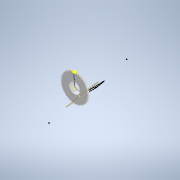
# Autodesk Inventor part: BigGear54T
Saved by Autodesk Inventor 2022 (Build 260153070, 153G)
## iProperties
Created: 2021-11-03
Part Number: BigGear54T
Material: Generic
Document SubType Name: Modeling
Designer: a laptop
Density: 1 g/cm^3
Appearance: Default
Author: a laptop
Autodesk Inventor part; units mm, degrees
ref_plane "YZ Plane" through (0, 0, 0) normal (1, 0, 0) x (0, 1, 0)
ref_plane "XZ Plane" through (0, 0, 0) normal (0, 1, 0) x (-1, 0, 0)
ref_plane "XY Plane" through (0, 0, 0) normal (0, 0, 1) x (1, 0, 0)
sketch "Sketch1" plane through (0, 0, 0) normal (0, 0, 1) x (1, 0, 0)
  spline S0 degree 3 poles (-1.174, 28.63) (-1.0927, 28.4349) (-0.9299, 28.0448) (-0.6964, 27.4567) (-0.6845, 26.9812) (-0.5323, 26.7628) (-0.4495, 26.6948) (-0.2625, 26.656) (0, 26.6828) (0.2625, 26.656) (0.4495, 26.6948) (0.5323, 26.7628) (0.6845, 26.9812) (0.6964, 27.4567) (0.9299, 28.0448) (1.0927, 28.4349) (1.174, 28.63) knots 0 0 0 0 0.063388 0.126771 0.190074 0.197992 0.205919 0.221604 0.2533 0.284997 0.300682 0.308609 0.316526 0.37983 0.443213 0.506601 0.506601 0.506601 0.506601
  circle A0 centre (0, 0) radius 26.6721 construction
  circle A1 centre (0, 0) radius 26.5898 construction
  circle A2 centre (0, 0) radius 27 construction
  circle A3 centre (0, 0) radius 28.654
  point P0 (-0.9317, 28.0443)
  point P1 (-0.7324, 27.4425)
  point P2 (-0.5764, 26.829)
  point P3 (-0.5295, 26.7652)
  point P4 (-0.4679, 26.7154)
  point P5 (-0.317, 26.6726)
  point P6 (0, 26.6721)
  point P7 (0.317, 26.6726)
  point P8 (0.4679, 26.7154)
  point P9 (0.5295, 26.7652)
  point P10 (0.5764, 26.829)
  point P11 (0.7324, 27.4425)
  point P12 (0.9317, 28.0443)
  constraints: 4 centre point, 2 point on circle, 35 other
extrude "Extrusion1" add sketch "Sketch1" against normal blind 3
extrude "Extrusion2" cut sketch "Sketch1" against normal blind 10 contours A3 S0 picked at (-0.134, 28.0575)
pattern_circular "Circular Pattern1" count 54 over 360 about axis through (0, 0, 0) along (0, 0, -1) of "Extrusion2"
sketch "Sketch2" plane through (0, 0, 0) normal (0, 0, 1) x (1, 0, 0)
  spline S0 degree 3 poles (-1.174, 28.63) (-1.0927, 28.4349) (-0.9299, 28.0448) (-0.6964, 27.4567) (-0.6845, 26.9812) (-0.5323, 26.7628) (-0.4495, 26.6948) (-0.2625, 26.656) (0, 26.6828) (0.2625, 26.656) (0.4495, 26.6948) (0.5323, 26.7628) (0.6845, 26.9812) (0.6964, 27.4567) (0.9299, 28.0448) (1.0927, 28.4349) (1.174, 28.63) knots 0 0 0 0 0.063388 0.126771 0.190074 0.197992 0.205919 0.221604 0.2533 0.284997 0.300682 0.308609 0.316526 0.37983 0.443213 0.506601 0.506601 0.506601 0.506601 projected
  arc A0 (-1.174, 28.63) -> (-2.1576, 28.5727) centre (0, 0) ccw projected
  line L0 (-2.1576, 28.5727) -> (-1.6658, 28.6013) construction
  arc A1 (2.1576, 28.5727) -> (1.174, 28.63) centre (0, 0) ccw projected
  line L1 (-1.174, 28.63) -> (0, 28.63) construction
  line L2 (-1.6658, 28.6013) -> (0, 0) construction
  line L3 (0, 28.63) -> (0, 0) construction
  line L4 (0, 28.63) -> (1.174, 28.63) construction
  line L5 (-1.6658, 28.6013) -> (-1.174, 28.63) construction
  constraints: 12 end point, 3 perpendicular, 2 horizontal, 1 coincident, 1 collinear, 1 other
sketch "Sketch3" plane through (0, 0, 0) normal (0, 0, 1) x (1, 0, 0)
  circle A0 centre (0, 0) radius 11.05
  circle A1 centre (0, 0) radius 14.05
  dimension "d7" = 22.1
  dimension "d8" = 3
  constraints: 2 centre point, 2 coincident
  measures "d7" diameter of A0
  measures "d8" radial gap between concentric circles of A1 A0
extrude "Extrusion3" add sketch "Sketch3" against normal blind 9.5
sketch "Sketch4" plane through (0, 0, -9.5) normal (0, 0, -1) x (-1, 0, 0)
  circle A0 centre (0, 0) radius 14.05 projected
  circle A1 centre (0, 0) radius 9.3
  circle A2 centre (0, 0) radius 11.05 construction
  dimension "d11" = 1.75
  constraints: 1 centre point, 1 coincident
  measures "d11" radial gap between concentric circles of A2 A1
extrude "Extrusion4" add sketch "Sketch4" along normal blind 1.5
extrude "Extrusion5" cut sketch "Sketch3" against normal blind 3 contours A0
ref_plane "Work Plane1" through (26.7535, 10.2617, 0) normal (0.7699292, -0.6381293, 0) x (0.6381293, 0.7699292, 0)
sketch "Sketch5" plane through (26.7535, 10.2617, 0) normal (0.7699292, -0.6381293, 0) x (0.6381293, 0.7699292, 0)
  line L0 (-10.923, -3) -> (-39.023, -3) projected
  line L1 (-24.973, -3) -> (-24.973, -43.285) construction
  line L2 (-12.973, -3) -> (-12.973, -16.8196)
  circle A0 centre (-13.603, -40.285) radius 1.5
  circle A1 centre (-13.603, -40.285) radius 3
  arc A2 (-12.973, -16.8196) -> (-10.6636, -39.6851) centre (101.378, -16.8196) ccw
  line L3 (-13.603, -43.285) -> (-24.973, -43.285)
  line L4 (-36.973, -3) -> (-36.973, -16.8196)
  circle A3 centre (-36.343, -40.285) radius 1.5
  circle A4 centre (-36.343, -40.285) radius 3
  arc A5 (-39.2824, -39.6851) -> (-36.973, -16.8196) centre (-151.3239, -16.8196) ccw
  line L5 (-36.343, -43.285) -> (-24.973, -43.285)
  point P0 (-24.973, 0)
  dimension "d16" = 3
  dimension "d17" = 1.5
  dimension "d18" = 12
  dimension "d19" = 26.4654
  constraints: 10 end point, 8 point on circle, 7 symmetric about line, 6 centre point, 3 tangent, 2 coincident, 2 vertical, 1 horizontal, 1 midpoint, 1 point on line, 4 other
  measures "d16" diameter of A0
  measures "d17" radial gap between concentric circles of A0 A1
  measures "d18" distance between parallel lines of L1 L2
  measures "d19" distance from line of L3 L2.end
equation "\"d0\" = FaceWidth"
equation "\"Module\" = 1"
equation "\"PressureAngle\" = 10deg"
equation "\"UnitProfileClearance\" = 0.25"
equation "\"UnitRoundRadius\" = 0.3025"
equation "\"HeadDiameter\" = 57.30803"
equation "\"RootDiameter\" = 53.34411"
equation "\"BaseDiameter\" = 53.17962"
equation "\"PitchDiameter\" = 54"
equation "\"FaceWidth\" = 3"
equation "\"HelixAngle\" = 0"
equation "\"UnitCorrection\" = 0.922054"
equation "\"UnitAddendumModification\" = 0.268038"
equation "\"CircularPitch\" = 3.141593"
equation "\"UnitBacklashShift\" = 0"
equation "\"TotalToolShift\" = 0.92205"
equation "\"IsInternal\" = 0"
body "Solid1"
